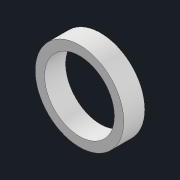
# Autodesk Inventor part: 4.5mm 0.5in Hex Spacer
Saved by Autodesk Inventor 2022 (Build 260153000, 153)
## iProperties
Created: 2022-09-24
Part Number: 4.5mm 0.5in Hex Spacer
Material: Generic
Document SubType Name: Modeling
Designer: robpl
Density: 1 g/cm^3
Appearance: Default
Author: robpl
Autodesk Inventor part; units mm, degrees
ref_plane "YZ Plane" through (0, 0, 0) normal (1, 0, 0) x (0, 1, 0)
ref_plane "XZ Plane" through (0, 0, 0) normal (0, 1, 0) x (-1, 0, 0)
ref_plane "XY Plane" through (0, 0, 0) normal (0, 0, 1) x (1, 0, 0)
sketch "Sketch1" plane through (0, 0, 0) normal (0, 0, 1) x (1, 0, 0)
  circle A0 centre (0, 0) radius 7.5
  circle A1 centre (0, 0) radius 9.5
  dimension "d0" = 15
  dimension "d1" = 19
  constraints: 2 centre point, 2 coincident
  measures "d0" diameter of A0
  measures "d1" diameter of A1
extrude "Extrusion1" add sketch "Sketch1" along normal blind 4.5
body "Solid1"
